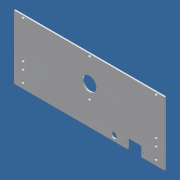
# Autodesk Inventor part: J001400
Saved by Autodesk Inventor 2012 SP2 (Build 160219200, 219)
## iProperties
Created: 2012-06-04
Part Number: J001400
Material: ALUMINUM, 6061-T651
Vendor: HHMI: JFRC - ID&F
Document SubType Name: Modeling
Designer: NEGRASHOVI
Density: 2.7 g/cm^3
Project: P-51601
Mass: 380.58 g
Surface Area: 928.375 cm^2
Volume: 140.956 cm^3
Description: BACK PANEL
RuleStatus: InUse
AfterDocSave0: file://Part Number Cleaner
LAB/DEPT: GONEN (LAB)
REQUESTING SCIENTIST: GONEN, TAMIR
SURFACE ROUGHNESS: 32 Ra
DESIGN DEPARTMENT: HHMI: JFRC - ID&F
SPECIAL FINISH: ANODIZE PER MIL-A-8625F, TYPE II, CLASS 2 (BLACK)
ALTERED ITEM PART NUMBER: N/A
ALTERED ITEM VENDOR: N/A
ALTERED ITEM DESCRIPTION: N/A
Author: NEGRASHOVI
Revision Number: -
Autodesk Inventor part; units mm, degrees
ref_plane "YZ Plane" through (0, 0, 0) normal (1, 0, 0) x (0, 1, 0)
ref_plane "XZ Plane" through (0, 0, 0) normal (0, 1, 0) x (-1, 0, 0)
ref_plane "XY Plane" through (0, 0, 0) normal (0, 0, 1) x (1, 0, 0)
sketch "Sketch1" plane through (0, 0, 0) normal (0, 0, 1) x (1, 0, 0)
  line L0 (-165.1, 69.85) -> (165.1, 69.85)
  line L1 (165.1, 69.85) -> (165.1, -69.85)
  line L2 (165.1, -69.85) -> (-165.1, -69.85)
  line L3 (-165.1, -69.85) -> (-165.1, 69.85)
  point P0 (0, 0)
  dimension "d0" = 139.7
  dimension "d1" = 330.2
  dimension "d2" = 69.85
  dimension "d3" = 165.1
  constraints: 8 end point, 2 parallel, 1 horizontal, 1 perpendicular
  measures "d0" distance of L0.end L1.end
  measures "d1" distance of L0.start L0.end
  measures "d2" distance from line of point (0, 0) L0
  measures "d3" distance from line of L1 point (0, 0)
extrude "Extrusion1" add sketch "Sketch1" along normal blind 3.175
sketch "Sketch4" plane through (0, 0, 3.175) normal (0, 0, 1) x (1, 0, 0)
  line L0 (-165.1, 69.85) -> (165.1, 69.85) projected
  line L1 (-165.1, -69.85) -> (-165.1, 69.85) projected
  line L2 (165.1, -69.85) -> (-165.1, -69.85) projected
  line L3 (165.1, 69.85) -> (165.1, -69.85) projected
  line L4 (-165.1, -15.875) -> (165.1, -15.875) construction
  line L5 (0, 69.85) -> (0, -69.85) construction
  line L6 (-146.05, 69.85) -> (-146.05, -69.85) construction
  line L7 (-165.1, 66.675) -> (165.1, 66.675) construction
  point P0 (0, 0)
  point P1 (-146.05, -15.875)
  point P2 (146.05, -15.875)
  point P3 (0, -15.875)
  point P4 (-146.05, -31.75)
  point P5 (-146.05, -57.15)
  point P6 (146.05, -31.75)
  point P7 (146.05, -57.15)
  point P8 (0, 66.675)
  point P9 (-146.05, 66.675)
  point P10 (146.05, 66.675)
  dimension "d24" = 85.725
  dimension "d49" = 12.7
  dimension "d50" = 25.4
  dimension "d90" = 3.175
  dimension "d92" = 146.05
  constraints: 15 point on line, 8 end point, 4 midpoint, 4 symmetric about line, 2 horizontal, 1 vertical
  measures "d24" distance between parallel lines of L4 L0
  measures "d49" distance from line of point (-146.05, -57.15) L2
  measures "d50" distance of point (-146.05, -31.75) point (-146.05, -57.15)
  measures "d90" distance between parallel lines of L0 L7
  measures "d92" distance between parallel lines of L6 L5
hole "Hole3" at (-146.05, -15.875, 3.175) at (146.05, -15.875, 3.175) at (0, -15.875, 3.175) at (-146.05, -31.75, 3.175) at (-146.05, -57.15, 3.175) at (146.05, -31.75, 3.175) at (146.05, -57.15, 3.175) at (-146.05, 66.675, 3.175) at (146.05, 66.675, 3.175) at (0, 66.675, 3.175) direction (0, 0, -1) diameter 3.81 end through all countersink diameter 7.0866 countersink angle 82 clearance for "Flat Head Machine Screw (82)" size "#6" standard "Ansi Unified Screw Threads"
sketch "Sketch7" plane through (0, 0, 3.175) normal (0, 0, 1) x (1, 0, 0)
  line L0 (0, -97.79) -> (0, 97.79) construction
  line L1 (-165.1, 69.85) -> (165.1, 69.85) projected
  point P0 (0, 0)
  point P1 (0, 12.7)
  dimension "d51" = 57.15
  constraints: 1 point on line
  measures "d51" distance from line of point (0, 12.7) L1
hole "Hole5" at (0, 12.7, 3.175) direction (0, 0, -1) diameter 30.9563 end through all
sketch "Sketch8" plane through (0, 0, 3.175) normal (0, 0, 1) x (1, 0, 0)
  line L0 (165.1, -69.85) -> (-165.1, -69.85) projected
  line L1 (83.82, -69.85) -> (114.3, -69.85)
  line L2 (114.3, -69.85) -> (114.3, -48.26)
  line L3 (114.3, -48.26) -> (83.82, -48.26)
  line L4 (83.82, -48.26) -> (83.82, -69.85)
  line L5 (165.1, 69.85) -> (165.1, -69.85) projected
  line L6 (99.06, -48.26) -> (99.06, -69.85) construction
  point P0 (0, 0)
  point P1 (79.0575, -58.42)
  point P2 (119.0625, -58.42)
  point P3 (53.6575, -58.42)
  dimension "d59" = 30.48
  dimension "d60" = 21.59
  dimension "d61" = 50.8
  dimension "d62" = 40.005
  dimension "d63" = 11.43
  dimension "d81" = 25.4
  dimension "d82" = 11.43
  constraints: 10 end point, 2 midpoint, 2 parallel, 1 horizontal, 1 perpendicular, 1 point on line, 1 symmetric about line
  measures "d59" distance of L2.end L3.end
  measures "d60" distance of L1.end L2.end
  measures "d61" distance between parallel lines of L5 L2
  measures "d62" distance of point (119.062, -58.42) point (79.057, -58.42)
  measures "d63" distance from line of point (119.062, -58.42) L0
  measures "d81" distance of point (53.657, -58.42) point (79.057, -58.42)
  measures "d82" distance from line of point (53.657, -58.42) L0
extrude "Extrusion3" cut sketch "Sketch8" against normal up to next
hole "Hole6" at (79.0575, -58.42, 3.175) at (119.0625, -58.42, 3.175) direction (0, 0, -1) diameter 2.159 end through all
hole "Hole8" at (53.6575, -58.42, 3.175) direction (0, 0, -1) diameter 12.7 end through all
equation "\"d2\" = 0.5 * d0"
equation "\"d3\" = 0.5 * d1"
equation "\"d82\" = d63"
body "Solid1"
